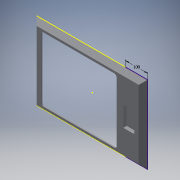
# Autodesk Inventor part: SitzFläche
Saved by Autodesk Inventor 2018 (Build 220112000, 112)
## iProperties
Created: 2019-02-06
Part Number: SitzFläche
Material: Generisch
Document SubType Name: Modeling
Designer: Lolob
Density: 1 g/cm^3
Appearance: Vorgabe
Author: Lolob
Autodesk Inventor part; units mm, degrees
ref_plane "YZ Plane" through (0, 0, 0) normal (1, 0, 0) x (0, 1, 0)
ref_plane "XZ Plane" through (0, 0, 0) normal (0, 1, 0) x (-1, 0, 0)
ref_plane "XY Plane" through (0, 0, 0) normal (0, 0, 1) x (1, 0, 0)
sketch "Skizze1" plane through (0, 0, 0) normal (0, 1, 0) x (-1, 0, 0)
  line L0 (350, 0) -> (-350, 0) projected
  line L1 (0, -245) -> (0, 245) projected
  line L2 (250, 175) -> (-250, 175)
  line L3 (-250, 175) -> (-250, -175)
  line L4 (-250, -175) -> (250, -175)
  line L5 (250, -175) -> (250, 175)
  point P0 (0, 0)
  dimension "d0" = 350
  dimension "d1" = 500
  constraints: 8 end point, 2 parallel, 1 horizontal, 1 perpendicular, 2 other
  measures "d0" distance of L2.end L3.end
  measures "d1" distance of L2.start L2.end
extrude "Extrusion1" add sketch "Skizze1" along normal blind 20
chamfer "Fase1" distance 20 angle 45 4 edges at (-250, 0, 0) (0, 0, 175) (250, 0, 0) (0, 0, -175)
sketch "Skizze2" plane through (0, 20, 0) normal (0, 1, 0) x (1, 0, 0)
  line L0 (250, -175) -> (250, 175) projected
  line L1 (250, 175) -> (-250, 175) projected
  line L2 (-250, -175) -> (250, -175) projected
  line L3 (250, 175) -> (150, 175)
  line L4 (150, 175) -> (150, -175)
  line L5 (150, -175) -> (250, -175)
  line L6 (250, -175) -> (250, 175)
  point P0 (0, 0)
  dimension "d7" = 100
  constraints: 8 end point, 2 parallel, 1 horizontal, 1 perpendicular, 1 point on line
  measures "d7" distance of L5.end L4.end
sketch "Skizze7" plane through (0, 20, 0) normal (0, 1, 0) x (1, 0, 0)
  line L0 (-250, -175) -> (250, -175) projected
  line L1 (250, -175) -> (250, 175) projected
  line L2 (250, 175) -> (-250, 175) projected
  line L3 (-250, 175) -> (-250, -175) projected
  line L4 (-350, 261.6691) -> (350, 261.6691)
  line L5 (-220, -165) -> (140, -165)
  line L6 (150, -155) -> (150, 155)
  line L7 (140, 165) -> (-220, 165)
  line L8 (-230, 155) -> (-230, -155)
  arc A0 (-230, -155) -> (-220, -165) centre (-220, -155) ccw
  arc A1 (-220, 165) -> (-230, 155) centre (-220, 155) ccw
  arc A2 (150, 155) -> (140, 165) centre (140, 155) ccw
  arc A3 (140, -165) -> (150, -155) centre (140, -155) ccw
  point P0 (0, 0)
  point P1 (458.9826, 261.6691)
  point P2 (-230, -165)
  point P3 (150, 165)
  point P4 (150, -165)
  point P5 (-230, 165)
  dimension "d35" = 380
  dimension "d36" = 330
  dimension "d37" = 20
  dimension "d38" = 10
  dimension "d41" = 10
  constraints: 10 end point, 8 point on circle, 8 point on line, 8 tangent, 4 centre point, 3 equal radius, 2 horizontal, 2 parallel, 1 perpendicular, 3 other
  measures "d35" distance of point (-230, -165) point (150, -165)
  measures "d36" distance of point (150, -165) point (150, 165)
  measures "d37" distance between parallel lines of L3 L8
  measures "d38" distance between parallel lines of L0 L5
  measures "d41" radius of A0
extrude "Extrusion6" cut sketch "Skizze7" against normal blind 10 contours A0 L8 A1 L7 A2 L6 A3 L5
sketch "Skizze6" plane through (0, 0, 0) normal (0, -1, 0) x (1, 0, 0)
  line L0 (120, 135) -> (120, -135) projected
  line L1 (230, 155) -> (230, -155) projected
  line L2 (-350, 0) -> (350, 0) projected
  line L3 (160, 42.534) -> (210, 42.534)
  line L4 (210, 42.534) -> (210, -47.466)
  line L5 (210, -47.466) -> (160, -47.466)
  line L6 (160, -47.466) -> (160, 42.534)
  point P0 (0, 0)
  point P1 (125, 150)
  point P2 (125, -150)
  dimension "d23" = 50
  dimension "d24" = 90
  dimension "d25" = 20
  constraints: 8 end point, 2 parallel, 1 horizontal, 1 perpendicular, 1 other
  measures "d23" distance of L3.start L3.end
  measures "d24" distance of L3.end L4.end
  measures "d25" distance between parallel lines of L1 L4
extrude "Extrusion5" cut sketch "Skizze6" against normal blind 15
fillet "Rundung1" radius 4 4 edges at (160, 7.5, 42.534) (210, 7.5, 42.534) (210, 7.5, -47.466) (160, 7.5, -47.466)
sketch "Skizze8" plane through (0, 10, 0) normal (0, 1, 0) x (1, 0, 0)
  line L0 (-220, -165) -> (140, -165) projected
  arc A0 (140, -165) -> (150, -155) centre (140, -155) ccw projected
  line L1 (150, 155) -> (150, -155) projected
  arc A1 (150, 155) -> (140, 165) centre (140, 155) ccw projected
  line L2 (140, 165) -> (-220, 165) projected
  arc A2 (-220, 165) -> (-230, 155) centre (-220, 155) ccw projected
  line L3 (-230, -155) -> (-230, 155) projected
  arc A3 (-230, -155) -> (-220, -165) centre (-220, -155) ccw projected
  line L4 (-220, 165) -> (140, 165) projected
  line L5 (-210, -155) -> (130, -155)
  line L6 (140, -145) -> (140, 145)
  line L7 (130, 155) -> (-210, 155)
  line L8 (-220, 145) -> (-220, -145)
  line L9 (230, 155) -> (-230, 155) projected
  arc A4 (-220, -145) -> (-210, -155) centre (-210, -145) ccw
  arc A5 (130, -155) -> (140, -145) centre (130, -145) ccw
  arc A6 (140, 145) -> (130, 155) centre (130, 145) ccw
  arc A7 (-210, 155) -> (-220, 145) centre (-210, 145) ccw
  point P0 (0, 0)
  dimension "d42" = 10
  dimension "d43" = 10
  dimension "d45" = 10
  dimension "d46" = 10
  dimension "d52" = 10
  constraints: 8 end point, 8 point on circle, 8 tangent, 4 centre point, 3 equal radius, 2 parallel, 1 horizontal, 1 perpendicular
  measures "d42" distance between parallel lines of L0 L5
  measures "d43" distance between parallel lines of L3 L8
  measures "d45" distance between parallel lines of L1 L6
  measures "d46" radius of A4
  measures "d52" distance between parallel lines of L2 L7
extrude "Extrusion7" cut sketch "Skizze8" against normal blind 5 contours L7 A6 L6 A5 L5 A4 L8 A7
sketch "Skizze9" plane through (0, 5, 0) normal (0, 1, 0) x (1, 0, 0)
  line L0 (130, -155) -> (-210, -155) projected
  arc A0 (130, -155) -> (140, -145) centre (130, -145) ccw projected
  line L1 (140, 145) -> (140, -145) projected
  arc A1 (140, 145) -> (130, 155) centre (130, 145) ccw projected
  line L2 (-210, 155) -> (130, 155) projected
  arc A2 (-210, 155) -> (-220, 145) centre (-210, 145) ccw projected
  line L3 (-220, -145) -> (-220, 145) projected
  arc A3 (-220, -145) -> (-210, -155) centre (-210, -145) ccw projected
  line L4 (-200, -145) -> (120, -145)
  line L5 (130, -135) -> (130, 135)
  line L6 (120, 145) -> (-200, 145)
  line L7 (-210, 135) -> (-210, -135)
  arc A4 (-210, -135) -> (-200, -145) centre (-200, -135) ccw
  arc A5 (-200, 145) -> (-210, 135) centre (-200, 135) ccw
  arc A6 (130, 135) -> (120, 145) centre (120, 135) ccw
  arc A7 (120, -145) -> (130, -135) centre (120, -135) ccw
  point P0 (0, 0)
  dimension "d49" = 10
  constraints: 8 end point, 8 point on circle, 8 tangent, 4 centre point, 4 point on line, 3 equal radius, 2 parallel, 1 horizontal, 1 perpendicular
  measures "d49" radius of A4
extrude "Extrusion8" cut sketch "Skizze9" against normal blind 5 contours A4 L7 A5 L6 A6 L5 A7 L4
